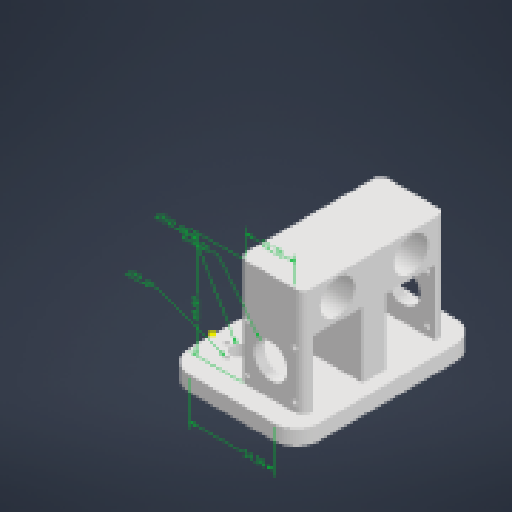
# Autodesk Inventor part: midle part
Saved by Autodesk Inventor 2024.2 (Build 282272000, 272)
## iProperties
Created: 2024-03-08
Part Number: midle part
Material: Generic
Document SubType Name: Modeling
Designer: seifs
Density: 1 g/cm^3
Appearance: Default
Author: seifs
Autodesk Inventor part; units mm, degrees
ref_plane "YZ Plane" through (0, 0, 0) normal (1, 0, 0) x (0, 1, 0)
ref_plane "XZ Plane" through (0, 0, 0) normal (0, 1, 0) x (-1, 0, 0)
ref_plane "XY Plane" through (0, 0, 0) normal (0, 0, 1) x (1, 0, 0)
sketch "Sketch1" plane through (0, 0, 0) normal (0, 1, 0) x (-1, 0, 0)
  line L0 (-14.9957, -29.7286) -> (-35, -29.7286)
  line L1 (-35.0352, 29.7286) -> (-15.013, 29.7286)
  line L2 (-50, 0) -> (-17.5, 0) construction
  circle A0 centre (-17.5, 0) radius 8 construction
  circle A1 centre (-9.5, 0) radius 1.6
  circle A2 centre (-25.5, 0) radius 1.6
  circle A3 centre (-17.5, -8) radius 1.6
  circle A4 centre (-17.5, 8) radius 1.6
  circle A5 centre (-17.5, 0) radius 5.1
  line L3 (-35, -29.7286) -> (-70, -29.7286)
  line L4 (-70, 29.7286) -> (-35.0352, 29.7286)
  line L5 (-85, 0.2714) -> (-85, 14.7286)
  line L6 (-85, 0.2714) -> (-85, -14.7286)
  arc A6 (-70, 29.7286) -> (-85, 14.7286) centre (-70, 14.7286) ccw
  line L7 (0, 0) -> (0.0043, -14.7242)
  line L8 (0, 0) -> (-0.013, 14.7419)
  arc A7 (-0.013, 14.7419) -> (-15.013, 29.7286) centre (-15.013, 14.7286) ccw
  line L9 (-85, -14.7286) -> (-85, -29.7286)
  line L10 (-85, -29.7286) -> (-70, -29.7286)
  line L11 (0.0043, -14.7242) -> (0.0043, -29.7286)
  line L12 (0.0043, -29.7286) -> (-14.9957, -29.7286)
  point P0 (-95, -29.7286)
  dimension "d3" = 32.5
  dimension "d5" = 16
  dimension "d6" = 3.2
  dimension "d7" = 3.2
  dimension "d8" = 3.2
  dimension "d9" = 3.2
  dimension "d10" = 10.2
  dimension "d20" = 60
  constraints: 26 end point, 8 centre point, 8 point on circle, 4 tangent, 3 horizontal, 3 vertical, 2 coincident, 2 perpendicular, 2 point on line, 1 parallel
  measures "d3" distance of L2.start L2.end
  measures "d5" diameter of A0
  measures "d6" diameter of A1
  measures "d7" diameter of A2
  measures "d8" diameter of A3
  measures "d9" diameter of A4
  measures "d10" diameter of A5
  measures "d20" distance of L0.end point (-95, -29.729)
extrude "Extrusion1" add sketch "Sketch1" along normal blind 10
sketch "Sketch3" plane through (0, 10, 0) normal (0, 1, 0) x (1, 0, 0)
  point P0 (0, 0)
sketch "Sketch4" plane through (0, 10, 0) normal (0, 1, 0) x (1, 0, 0)
  circle A0 centre (25.5, 0) radius 1.6 projected
  line L0 (25.5, 0) -> (35.5, 0) construction
  line L1 (85, 29.7286) -> (-0.0043, 29.7286) projected
  line L2 (34.1, 29.7286) -> (34.1, 0) construction
  line L3 (34.1, -10.2714) -> (76.4, -10.2714)
  line L4 (76.4, -16.7714) -> (34.1, -16.7714)
  line L5 (27.1, 0) -> (34.1, 0)
  line L6 (34.1, 0) -> (34.1, -16.7714)
  line L7 (76.4, -10.2714) -> (76.4, -16.7714)
  point P0 (0, 0)
  point P1 (80, 30)
  point P2 (-35.0174, 29.7286)
  point P3 (67.8, 30)
  point P4 (70, 29.7286)
  point P5 (14.9957, 29.7286)
  point P6 (-0.0043, 29.7286)
  dimension "d22" = 10
  dimension "d23" = 40
  dimension "d25" = 6.5
  dimension "d47" = 7
  dimension "d49" = 42.3
  constraints: 14 end point, 3 perpendicular, 3 point on line, 2 horizontal, 1 horizontal alignment, 1 vertical, 3 other
  measures "d22" distance of L0.start L0.end
  measures "d23" distance of L2.start L3.start
  measures "d25" distance of L3.end L4.start
  measures "d47" distance of L2.end L5.start
  measures "d49" distance of L3.start L3.end
extrude "Extrusion3" add sketch "Sketch4" along normal blind 70 contours L3 L7 L4 L6
sketch "Sketch5" plane through (37.7, 10, 16.7714) normal (0, 0, 1) x (1, 0, 0)
  line L0 (-3.6, 0) -> (38.7, 0) construction
  line L1 (17.55, 0) -> (17.55, 21.15) construction
  circle A0 centre (17.55, 21.15) radius 11
  line L2 (17.55, 21.15) -> (17.55, 36.65) construction
  line L3 (17.55, 36.65) -> (2.05, 36.65) construction
  line L4 (2.05, 36.65) -> (2.05, 5.65) construction
  line L5 (2.05, 5.65) -> (33.05, 5.65) construction
  line L6 (33.05, 5.65) -> (33.05, 36.65) construction
  circle A1 centre (2.05, 36.65) radius 1.5
  circle A2 centre (33.05, 36.65) radius 1.5
  circle A3 centre (33.05, 5.65) radius 1.5
  circle A4 centre (2.05, 5.65) radius 1.5
  point P0 (-37.7, -10)
  point P1 (0, 0)
  point P2 (42.3, 0)
  dimension "d28" = 21.15
  dimension "d29" = 22
  dimension "d30" = 15.5
  dimension "d31" = 15.5
  dimension "d32" = 31
  dimension "d33" = 31
  dimension "d34" = 3
  dimension "d35" = 3
  dimension "d36" = 3
  dimension "d37" = 3
  constraints: 12 end point, 5 centre point, 5 coincident, 3 perpendicular, 2 vertical, 1 midpoint, 1 parallel, 1 point on line
  measures "d28" distance of L1.start L1.end
  measures "d29" diameter of A0
  measures "d30" distance of L2.start L2.end
  measures "d31" distance of L2.end L3.end
  measures "d32" distance of L3.end L4.end
  measures "d33" distance of L4.end L5.end
  measures "d34" diameter of A1
  measures "d35" diameter of A2
  measures "d36" diameter of A3
  measures "d37" diameter of A4
extrude "Extrusion4" cut sketch "Sketch5" against normal blind 10.25
sketch "Sketch7" plane through (76.4, 10, 10.2714) normal (0, 0, -1) x (-1, 0, 0)
  line L0 (42.3, 43) -> (0, 43)
  line L1 (0, 70) -> (0, 43)
  line L2 (42.3, 70) -> (42.3, 43)
  line L3 (0, 70) -> (42.3, 70) projected
  line L4 (0, 70) -> (42.3, 70)
  point P0 (76.4, -10)
  point P1 (21.15, 43)
  dimension "d98" = 27
  constraints: 8 end point, 2 vertical, 1 collinear, 1 midpoint
  measures "d98" distance from line of point (21.15, 43) L3
extrude "Extrusion5" add sketch "Sketch7" along normal blind 40
sketch "Sketch8" plane through (76.4, 10, 16.7714) normal (1, 0, 0) x (0, 0, -1)
  line L0 (45.004, 44.6948) -> (22.504, 44.6948) construction
  circle A0 centre (22.5, 57) radius 11
  line L1 (6.5, 43) -> (46.5, 43) projected
  point P0 (16.7714, -10)
  dimension "d59" = 22.5
  dimension "d95" = 22
  dimension "d97" = 14
  constraints: 2 end point, 1 centre point, 1 horizontal
  measures "d59" distance of L0.start L0.end
  measures "d95" diameter of A0
  measures "d97" distance from line of L1 A0.centre
extrude "Extrusion6" cut sketch "Sketch8" against normal blind 30
sketch "Sketch9" plane through (0, 80, 0) normal (0, 1, 0) x (1, 0, 0)
  line L0 (40.1, 29.7286) -> (40.1, 23.7286) construction
  line L1 (76.4, -16.7714) -> (76.4, 29.7286) projected
  line L2 (34.1, -10.2714) -> (34.1, 29.7286) projected
  line L3 (76.4, 22.1286) -> (34.1, 22.1286)
  line L4 (34.1, 22.1286) -> (34.1, 29.7286)
  line L5 (34.1, 29.7286) -> (76.4, 29.7286)
  line L6 (76.4, 29.7286) -> (76.4, 22.1286)
  dimension "d64" = 6
  constraints: 10 end point, 2 parallel, 1 horizontal, 1 perpendicular, 1 point on line
  measures "d64" distance of L0.start L0.end
extrude "Extrusion7" add sketch "Sketch9" against normal blind 70
fillet "Face Fillet4" radius 5 1 edges at (76.4, 45, 16.7714)
fillet "Face Fillet5" radius 5 1 edges at (34.1, 45, 16.7714)
mirror "Mirror1" about plane through (55.25, 66.5, -29.7286) normal (0, 0, -1)
sketch "Sketch10" plane through (0, 10, 0) normal (0, 1, 0) x (1, 0, 0)
  circle A0 centre (17.5, 59.4572) radius 5.1 projected
  circle A1 centre (25.5, 59.4572) radius 1.6 projected
  circle A2 centre (17.5, 67.4572) radius 1.6 projected
  circle A3 centre (17.5, 51.4572) radius 1.6 projected
  circle A4 centre (9.5, 59.4572) radius 1.6 projected
  point P0 (0, 0)
extrude "Extrusion8" add sketch "Sketch10" against normal blind 10
body "Solid1"
